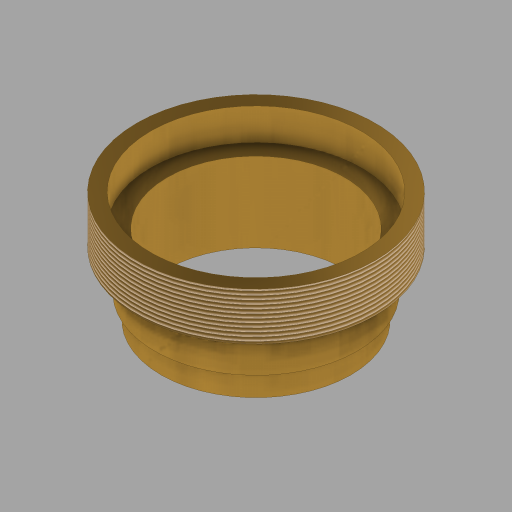
# Autodesk Inventor part: neck
Saved by Autodesk Inventor 2024 (Build 280153020, 153B)
## iProperties
Created: 2023-11-04
Part Number: neck
Material: Brass
Document SubType Name: Modeling
Designer: schanen
Density: 8.49 g/cm^3
Appearance: Brass - Polished
Mass: 138.614 g
Surface Area: 114.103 cm^2
Volume: 16.3653 cm^3
neck_thread_dia: 30.000 mm
neck_thread_len: 12.000 mm
neck_ir: 22.325 mm
Author: schanen
Autodesk Inventor part; units mm, degrees
ref_plane "YZ Plane" through (0, 0, 0) normal (1, 0, 0) x (0, 1, 0)
ref_plane "XZ Plane" through (0, 0, 0) normal (0, 1, 0) x (-1, 0, 0)
ref_plane "XY Plane" through (0, 0, 0) normal (0, 0, 1) x (1, 0, 0)
sketch "Sketch1" plane through (0, 0, 0) normal (0, 0, 1) x (1, 0, 0)
  line L0 (-22.325, 20) -> (-22.325, 0)
  line L1 (-22.325, 0) -> (-23.9, 0)
  line L2 (-23.9, 0) -> (-23.9, 6)
  line L3 (-23.9, 6) -> (-25.5, 6)
  line L4 (-25.5, 6) -> (-25.5, 16)
  line L5 (-25.5, 16) -> (-30, 16)
  line L6 (-30, 16) -> (-30, 28)
  line L7 (-30, 28) -> (-26.5, 28)
  line L8 (-26.5, 28) -> (-26.5, 20)
  line L9 (-26.5, 20) -> (-22.325, 20)
  line L10 (0, -5.6) -> (0, 33.6) projected
  point P0 (0, 0)
  dimension "d0" = 23.9
  dimension "neck_ir" = 22.325
  dimension "d4" = 8
  dimension "d5" = 6
  dimension "d7" = 10
  dimension "neck_thread_dia" = 30
  dimension "neck_thread_len" = 12
  dimension "d14" = 26.5
  dimension "d15" = 25.5
  constraints: 20 end point, 9 perpendicular, 1 horizontal alignment, 1 vertical
  measures "d0" distance from line of point (0, 0) L2
  measures "neck_ir" distance from line of point (0, 0) L0
  measures "d4" distance of L7.end L8.end
  measures "d5" distance of L1.end L2.end
  measures "d7" distance of L3.end L4.end
  measures "neck_thread_dia" distance from line of point (0, 0) L6
  measures "neck_thread_len" distance of L5.end L6.end
  measures "d14" distance between parallel lines of L10 L8
  measures "d15" distance from line of point (0, 0) L4
revolve "Revolution1" add sketch "Sketch1" angle 360 about axis through (0, -10, 0) along (0, 1, 0)
thread "Thread1" size "M60x1" class "6g" standard "ANSI Metric M Profile" full length
equation "\"d4\" = 2 * oring_dia"
equation "\"d14\" = 0.5 * oring_od"
equation "\"oring_diameter\" = 4"
equation "\"oring_dia\" = 4"
equation "\"oring_od\" = 53"
body "Solid1"
